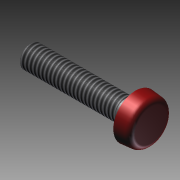
# Autodesk Inventor part: 205-S-AS
Saved by Autodesk Inventor 2011 SP1 (Build 150282100, 282)
## iProperties
Created: 2017-03-01
Part Number: 205-S-AS
Catalog Web Link: www.cadenas.de
Description: AS-SU-Andruckspindel
Vendor: DESTACO
Document SubType Name: Modeling
Designer: psAdmin
Manufacturer: DESTACO
Mass: 0.365209 g
Surface Area: 4.00024 cm^2
Volume: 0.365209 cm^3
Density: 1 g/cm^3
Category: PARTsolutions
Company: DESTACO
Title: 205-S-AS
Author: Cadenas PARTsolutions
Comments: Andruckspindel
PSOL_IDENT_0: {$CADENAS_DATA\23d-libs\destaco\destaco_gmbh\man_spann\horizontalspanner\standard\su_parts\andrucksp
PSOL_IDENT_1: indel_su.prj},159 {VTYP=3D},{NB=205-S-AS},{LINA=205-S-AS},{NN=AS-SU},{DATE=20.09.2016 07:53:12},{GEO
PSOL_IDENT_2: MDATE=08.12.2009 09:16:00},{VERSION=v1},{LINEID=20},{LINESUBID=-1},{WBVAR=}  {NB=205-S-AS},{LINA=205
PSOL_IDENT_3: -S-AS},{KT=DUMMY},{MODELL=205-S-AS},{SIZE=1},{MOD=1.000}
NN: AS-SU
NT: Andruckspindel
NB: 205-S-AS
NBSYN: $MODELL.
LINA: 205-S-AS
MODELL: 205-S-AS
SIZE: 1
MOD: 1.000
SUPPLIER: DESTACO
ARTICLENO: 205-S-AS
BOMINFO: 205-S-AS
CREATOR: CADENAS GmbH
Autodesk Inventor part; units mm, degrees
sketch "Skizze_1" plane through (0, 0, 0) normal (0, 1, 0) x (-1, 0, 0)
  line L0 (-22, 0) -> (0, 0)
  line L1 (0, 0) -> (0, -1.5705)
  line L2 (0, -1.5705) -> (-0.4295, -2)
  line L3 (-0.4295, -2) -> (-18.5, -2)
  line L4 (-18.5, -2) -> (-18.5, -1.5705)
  line L5 (-18.5, -1.5705) -> (-19.2, -1.5705)
  line L6 (-19.2, -1.5705) -> (-19.2, -4)
  line L7 (-19.2, -4) -> (-21.0872, -3.8349)
  arc A0 (-22, -2.8387) -> (-21.0872, -3.8349) centre (-21, -2.8387) ccw
  line L8 (-22, -2.8387) -> (-22, 0)
  line L9 (-22, 0) -> (0, 0)
  constraints: 20 end point, 2 point on circle, 1 centre point
revolve "Revolution1" add sketch "Skizze_1" angle 360 about axis through (22, 0, 0) along (1, 0, 0)
thread "Thread1" size "M4x0.7" class "6g" standard "ISO Metric profile" length 17.0705
ref_plane "AS_XY" through (10.92, 0, 0) normal (1, 0, 0) x (0, 0, -1)
ref_plane "AS_YZ" through (10.92, 0, 0) normal (0, 0, -1) x (0, 1, 0)
ref_plane "AS_ZX" through (10.92, 0, 0) normal (0, 1, 0) x (1, 0, 0)
body "Solid1"
